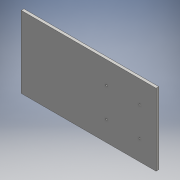
# Autodesk Inventor part: base
Saved by Autodesk Inventor 2016 (Build 200138000, 138)
## iProperties
Created: 2023-04-16
Part Number: base
Material: 常规
Document SubType Name: Modeling
Designer: Administrator
Density: 1 g/cm^3
Appearance: 默认
Author: Administrator
Autodesk Inventor part; units mm, degrees
ref_plane "YZ Plane" through (0, 0, 0) normal (1, 0, 0) x (0, 1, 0)
ref_plane "XZ Plane" through (0, 0, 0) normal (0, 1, 0) x (-1, 0, 0)
ref_plane "XY Plane" through (0, 0, 0) normal (0, 0, 1) x (1, 0, 0)
sketch "草图1" plane through (0, 0, 0) normal (0, 1, 0) x (-1, 0, 0)
  line L0 (0, 0) -> (-150, 0)
  line L1 (-150, 0) -> (-150, -80)
  line L2 (-150, -80) -> (0, -80)
  line L3 (0, -80) -> (0, 0)
  line L4 (-150, 0) -> (-132, 0)
  line L5 (-132, 0) -> (-132, -24.95)
  circle A0 centre (-132, -24.95) radius 1
  line L6 (-132, -24.95) -> (-132, -57.65)
  line L7 (-132, -57.65) -> (-95, -57.65)
  line L8 (-95, -57.65) -> (-95, -24.95)
  circle A1 centre (-95, -24.95) radius 1
  circle A2 centre (-95, -57.65) radius 1
  circle A3 centre (-132, -57.65) radius 1
  dimension "d0" = 150
  dimension "d1" = 80
  dimension "d2" = 18
  dimension "d3" = 24.95
  dimension "d4" = 2
  dimension "d5" = 32.7
  dimension "d6" = 37
  dimension "d7" = 32.7
  dimension "d8" = 2
  dimension "d9" = 2
  dimension "d10" = 2
  constraints: 18 end point, 4 centre point, 4 perpendicular, 2 parallel, 1 coincident, 1 horizontal, 1 point on line, 1 vertical
  measures "d0" distance of L2.end L1.end
  measures "d1" distance of L1.end L0.end
  measures "d2" distance of L0.end L4.end
  measures "d3" distance of L4.end L5.end
  measures "d4" diameter of A0
  measures "d5" distance of L6.start L6.end
  measures "d6" distance of L6.end L7.end
  measures "d7" distance of L7.end L8.end
  measures "d8" diameter of A1
  measures "d9" diameter of A2
  measures "d10" diameter of A3
extrude "拉伸1" add sketch "草图1" against normal blind 3
